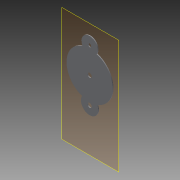
# Autodesk Inventor part: driveGearSupportLayer
Saved by Autodesk Inventor 2013 (Build 170138000, 138)
## iProperties
Created: 2014-07-02
Part Number: driveGearSupportLayer
Material: Generic
Document SubType Name: Modeling
Designer: Nano
Density: 1 g/cm^3
Author: Nano
Autodesk Inventor part; units mm, degrees
ref_plane "YZ Plane" through (0, 0, 0) normal (1, 0, 0) x (0, 1, 0)
ref_plane "XZ Plane" through (0, 0, 0) normal (0, 1, 0) x (-1, 0, 0)
ref_plane "XY Plane" through (0, 0, 0) normal (0, 0, 1) x (1, 0, 0)
ref_plane "Work Plane1" through (-99.6499, 20.9204, 0) normal (0, 0, 1) x (0.9625, -0.2713, 0)
sketch "Sketch1" plane through (-99.6499, 20.9204, 0) normal (0, 0, 1) x (0.9625, -0.2713, 0)
  arc A0 (85.2738, 81.502) -> (83.0074, 84.6783) centre (85.432, 84.0117) ccw construction
  circle A1 centre (88.0557, 106.0406) radius 3.175
  arc A2 (111.4983, 99.8389) -> (64.6131, 112.2422) centre (88.0557, 106.0406) ccw
  circle A3 centre (90.0577, 33.4227) radius 3.175 construction
  circle A4 centre (94.6835, -17.1663) radius 3.175 construction
  arc A5 (165.3065, -1.1832) -> (158.0816, 17.8159) centre (94.6835, -17.1663) ccw
  circle A6 centre (90.0577, 33.4227) radius 4.1833
  circle A7 centre (94.6835, -17.1663) radius 4.0324
  arc A8 (158.0816, 17.8159) -> (111.4983, 99.8389) centre (90.0577, 33.4227) ccw
  arc A9 (64.6131, 112.2422) -> (165.3065, -1.1832) centre (90.0577, 33.4227) ccw
  point P0 (101.5885, 6.8942)
  dimension "d0" = 6.35
  constraints: 8 point on circle, 7 centre point
  measures "d0" diameter of A1
extrude "Extrusion1" add sketch "Sketch1" along normal blind 1.5875
body "Solid1"
